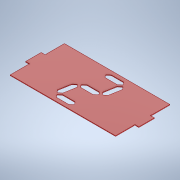
# Autodesk Inventor part: Cockpit_front_frame_cloth
Saved by Autodesk Inventor 2020 (Build 240168000, 168)
## iProperties
Created: 2022-04-01
Part Number: Cockpit_front_frame_cloth
Material: 一般
Document SubType Name: Modeling
Designer: Masato Kubotera
Density: 1 g/cm^3
Appearance: 滑らか - 赤
Author: Masato Kubotera
Autodesk Inventor part; units mm, degrees
ref_plane "XZ Plane" through (0, 0, 0) normal (0, 1, 0) x (-1, 0, 0)
ref_plane "XY Plane" through (0, 0, 0) normal (0, 0, 1) x (1, 0, 0)
derived "Cockpit_front_frame.ipt"
sketch "スケッチ2" plane through (0, 0, 0) normal (0, 1, 0) x (-1, 0, 0)
  line L0 (-28.5, -22.5) -> (88.5, -22.5) construction
  line L1 (88.5, -22.5) -> (88.5, -138.5)
  line L2 (88.5, -96) -> (-28.5, -96) construction
  line L3 (-28.5, -96) -> (-28.5, -22.5) construction
  line L4 (-28.5, -22.5) -> (88.5, -96) construction
  line L5 (88.5, -22.5) -> (-28.5, -96) construction
  line L6 (38.5, -101) -> (38.5, -133.5)
  line L7 (43.5, -138.5) -> (88.5, -138.5)
  line L8 (63.9, -63.85) -> (73.1, -63.85) construction
  line L9 (73.1, -63.85) -> (73.1, -77.65) construction
  line L10 (73.1, -77.65) -> (63.9, -77.65) construction
  line L11 (63.9, -77.65) -> (63.9, -63.85) construction
  line L12 (63.9, -63.85) -> (73.1, -77.65) construction
  line L13 (73.1, -63.85) -> (63.9, -77.65) construction
  line L14 (63.2, -63.2) -> (73.8, -63.2) construction
  line L15 (73.8, -63.2) -> (73.8, -78.3) construction
  line L16 (73.8, -78.3) -> (63.2, -78.3) construction
  line L17 (63.2, -78.3) -> (63.2, -63.2) construction
  line L18 (63.2, -63.2) -> (73.8, -78.3) construction
  line L19 (73.8, -63.2) -> (63.2, -78.3) construction
  line L20 (68.5, -63.2) -> (68.5, -78.3) construction
  line L21 (73.8, -70.75) -> (63.2, -70.75) construction
  line L22 (64.6349, -63.15) -> (72.3651, -63.15)
  line L23 (63.15, -64.6349) -> (63.15, -76.8651)
  line L24 (65.3349, -63.8) -> (71.6651, -63.8)
  line L25 (63.85, -65.2849) -> (63.85, -76.2151)
  arc A0 (64.6349, -63.15) -> (63.15, -64.6349) centre (63.8925, -63.8925) ccw
  arc A1 (65.3349, -63.8) -> (63.85, -65.2849) centre (64.5925, -64.5425) ccw
  arc A2 (73.85, -64.6349) -> (72.3651, -63.15) centre (73.1075, -63.8925) ccw
  arc A3 (73.15, -65.2849) -> (71.6651, -63.8) centre (72.4075, -64.5425) ccw
  line L26 (64.6349, -78.35) -> (72.3651, -78.35)
  line L27 (65.3349, -77.7) -> (71.6651, -77.7)
  arc A4 (63.85, -76.2151) -> (65.3349, -77.7) centre (64.5925, -76.9575) ccw
  arc A5 (63.15, -76.8651) -> (64.6349, -78.35) centre (63.8925, -77.6075) ccw
  arc A6 (72.3651, -78.35) -> (73.85, -76.8651) centre (73.1075, -77.6075) ccw
  arc A7 (71.6651, -77.7) -> (73.15, -76.2151) centre (72.4075, -76.9575) ccw
  line L28 (73.15, -65.2849) -> (73.15, -76.2151)
  line L29 (73.85, -64.6349) -> (73.85, -76.8651)
  line L30 (-23.5, -22.5) -> (-28.5, -27.5)
  line L31 (-28.5, -59.25) -> (88.5, -59.25) construction
  line L32 (30, -22.5) -> (30, -96) construction
  line L33 (-23.5, -96) -> (-28.5, -91)
  line L34 (-28.5, -27.5) -> (-28.5, -91)
  line L35 (-20.5, -24.5) -> (-25.5, -24.5) construction
  line L36 (-25.5, -24.5) -> (-25.5, -94) construction
  line L37 (-25.5, -94) -> (-20.5, -94) construction
  line L38 (-20.5, -94) -> (-20.5, -24.5) construction
  line L39 (-20.5, -24.5) -> (-25.5, -94) construction
  line L40 (-25.5, -24.5) -> (-20.5, -94) construction
  line L41 (-25.55, -46.7) -> (-20.45, -46.7)
  line L42 (-20.45, -46.7) -> (-20.45, -71.8)
  line L43 (-20.45, -71.8) -> (-25.55, -71.8)
  line L44 (-25.55, -71.8) -> (-25.55, -46.7)
  line L45 (-25.55, -46.7) -> (-20.45, -71.8) construction
  line L46 (-20.45, -46.7) -> (-25.55, -71.8) construction
  line L47 (-25.5, -46.75) -> (-20.5, -46.75) construction
  line L48 (-25.5, -71.75) -> (-20.5, -71.75) construction
  line L49 (-23, -24.5) -> (-23, -94) construction
  circle A8 centre (-23, -35) radius 3
  circle A9 centre (-23, -35) radius 1.6
  arc A10 (-24.0651, -46.7) -> (-25.55, -48.1849) centre (-24.8075, -47.4425) ccw
  arc A11 (-20.45, -48.1849) -> (-21.9349, -46.7) centre (-21.1925, -47.4425) ccw
  arc A12 (-25.55, -70.3151) -> (-24.0651, -71.8) centre (-24.8075, -71.0575) ccw
  arc A13 (-21.9349, -71.8) -> (-20.45, -70.3151) centre (-21.1925, -71.0575) ccw
  circle A14 centre (-23, -83.5) radius 3
  circle A15 centre (-23, -83.5) radius 1.6
  line L50 (33.5, -96) -> (38.5, -101)
  line L51 (-23.5, -96) -> (33.5, -96)
  line L52 (81, -42.5) -> (-20.5, -42.5) construction
  line L53 (-20.5, -42.5) -> (-20.5, -37.5) construction
  line L54 (-20.5, -37.5) -> (81, -37.5) construction
  line L55 (81, -37.5) -> (81, -42.5) construction
  line L56 (81, -42.5) -> (-20.5, -37.5) construction
  line L57 (-20.5, -42.5) -> (81, -37.5) construction
  line L58 (-20.5, -40) -> (81, -40) construction
  line L59 (30.25, -37.5) -> (30.25, -42.5) construction
  line L60 (5.25, -37.5) -> (5.25, -42.5) construction
  line L61 (55.3, -37.45) -> (5.2, -37.45)
  line L62 (5.2, -37.45) -> (5.2, -42.55)
  line L63 (5.2, -42.55) -> (55.3, -42.55)
  line L64 (55.3, -42.55) -> (55.3, -37.45)
  line L65 (55.3, -37.45) -> (5.2, -42.55) construction
  line L66 (5.2, -37.45) -> (55.3, -42.55) construction
  arc A16 (6.6849, -37.45) -> (5.2, -38.9349) centre (5.9425, -38.1925) ccw
  circle A17 centre (-2.25, -40) radius 3
  circle A18 centre (-2.25, -40) radius 1.6
  line L67 (55.25, -37.5) -> (55.25, -42.5) construction
  arc A19 (55.3, -38.9349) -> (53.8151, -37.45) centre (54.5575, -38.1925) ccw
  circle A20 centre (62.75, -40) radius 3
  circle A21 centre (62.75, -40) radius 1.6
  arc A22 (5.2, -41.0651) -> (6.6849, -42.55) centre (5.9425, -41.8075) ccw
  arc A23 (53.8151, -42.55) -> (55.3, -41.0651) centre (54.5575, -41.8075) ccw
  line L68 (-20.5, -89) -> (81, -89) construction
  line L69 (81, -89) -> (81, -94) construction
  line L70 (81, -94) -> (-20.5, -94) construction
  line L71 (-20.5, -94) -> (-20.5, -89) construction
  line L72 (-20.5, -89) -> (81, -94) construction
  line L73 (81, -89) -> (-20.5, -94) construction
  line L74 (-20.5, -91.5) -> (81, -91.5) construction
  line L75 (30.25, -89) -> (30.25, -94) construction
  line L76 (55.3, -91.55) -> (5.2, -91.55)
  line L77 (5.2, -91.55) -> (5.2, -88.95)
  line L78 (5.2, -88.95) -> (55.3, -88.95)
  line L79 (55.3, -88.95) -> (55.3, -91.55)
  line L80 (55.3, -91.55) -> (5.2, -88.95) construction
  line L81 (5.2, -91.55) -> (55.3, -88.95) construction
  line L82 (5.25, -89) -> (5.25, -91.5) construction
  line L83 (55.25, -89) -> (55.25, -91.5) construction
  line L84 (5.25, -90.25) -> (55.25, -90.25) construction
  arc A24 (7.3, -88.95) -> (5.2, -88.95) centre (6.25, -88.95) ccw
  arc A25 (55.3, -88.95) -> (53.2, -88.95) centre (54.25, -88.95) ccw
  arc A26 (5.2, -91.55) -> (7.3, -91.55) centre (6.25, -91.55) ccw
  arc A27 (53.2, -91.55) -> (55.3, -91.55) centre (54.25, -91.55) ccw
  circle A28 centre (-2.5, -91.5) radius 3
  circle A29 centre (-2.5, -91.5) radius 1.6
  circle A30 centre (62.5, -91.5) radius 3 construction
  circle A31 centre (62.5, -91.5) radius 1.6 construction
  line L85 (-23.5, -22.5) -> (63.7651, -22.5)
  line L86 (65.25, -21.0151) -> (65.25, -17.5)
  line L87 (65.25, -17.5) -> (73.25, -17.5)
  line L88 (73.25, -17.5) -> (73.25, -21.0151)
  line L89 (81, -22.5) -> (81, -17.5)
  line L90 (88.5, -22.5) -> (88.5, -20)
  line L91 (81, -17.5) -> (86, -17.5)
  line L92 (86, -17.5) -> (88.5, -20)
  line L93 (69.25, -17.5) -> (69.25, -22.5) construction
  arc A32 (63.7651, -22.5) -> (65.25, -21.0151) centre (64.5075, -21.7575) ccw
  arc A33 (73.25, -21.0151) -> (74.7349, -22.5) centre (73.9925, -21.7575) ccw
  arc A34 (79.5151, -22.5) -> (81, -21.0151) centre (80.2575, -21.7575) ccw
  line L94 (-15.5, -89) -> (-15.5, -69) construction
  line L95 (-15.5, -69) -> (64.5, -69) construction
  line L96 (64.5, -69) -> (64.5, -89) construction
  line L97 (45.5, -84) -> (-16.5, -84)
  line L98 (-18.5, -82) -> (-18.5, -63.3955)
  line L99 (-16.5, -61.3955) -> (45.5, -61.3955)
  line L100 (47.5, -63.3955) -> (47.5, -82)
  line L101 (47.5, -84) -> (-18.5, -61.3955) construction
  line L102 (-18.5, -84) -> (47.5, -61.3955) construction
  arc A35 (-16.5, -61.3955) -> (-18.5, -63.3955) centre (-16.5, -63.3955) ccw
  arc A36 (-18.5, -82) -> (-16.5, -84) centre (-16.5, -82) ccw
  arc A37 (45.5, -84) -> (47.5, -82) centre (45.5, -82) ccw
  arc A38 (47.5, -63.3955) -> (45.5, -61.3955) centre (45.5, -63.3955) ccw
  line L103 (38.5, -133.5) -> (43.5, -138.5)
  line L104 (46, -131) -> (41, -131) construction
  line L105 (41, -131) -> (41, -96) construction
  line L106 (41, -96) -> (46, -96) construction
  line L107 (46, -96) -> (46, -131) construction
  line L108 (46, -131) -> (41, -96) construction
  line L109 (41, -131) -> (46, -96) construction
  line L110 (43.5, -96) -> (43.5, -131) construction
  line L111 (41, -113.5) -> (46, -113.5) construction
  line L112 (43.5, -107.5) -> (46, -107.5) construction
  line L113 (43.45, -107.45) -> (46.05, -107.45)
  line L114 (46.05, -107.45) -> (46.05, -119.55)
  line L115 (46.05, -119.55) -> (43.45, -119.55)
  line L116 (43.45, -119.55) -> (43.45, -107.45)
  line L117 (43.45, -107.45) -> (46.05, -119.55) construction
  line L118 (46.05, -107.45) -> (43.45, -119.55) construction
  arc A39 (46.05, -109.55) -> (46.05, -107.45) centre (46.05, -108.5) ccw
  arc A40 (44.9349, -107.45) -> (43.45, -108.9349) centre (44.1925, -108.1925) ccw
  line L119 (43.5, -119.5) -> (46, -119.5) construction
  arc A41 (46.05, -119.55) -> (46.05, -117.45) centre (46.05, -118.5) ccw
  arc A42 (43.45, -118.0651) -> (44.9349, -119.55) centre (44.1925, -118.8075) ccw
  line L120 (44.75, -107.5) -> (44.75, -119.5) construction
  circle A43 centre (43.5, -125.5) radius 3 construction
  circle A44 centre (43.5, -125.5) radius 1.6 construction
  circle A45 centre (43.5, -101.5) radius 3
  circle A46 centre (43.5, -101.5) radius 1.6
  circle A47 centre (-13.5, -55) radius 2
  line L121 (41, -131) -> (79.8645, -131) construction
  line L122 (79.8645, -131) -> (79.8645, -136) construction
  line L123 (79.8645, -136) -> (41, -136) construction
  line L124 (41, -136) -> (41, -131) construction
  line L125 (41, -131) -> (79.8645, -136) construction
  line L126 (79.8645, -131) -> (41, -136) construction
  line L127 (41, -133.5) -> (79.8645, -133.5) construction
  line L128 (60.4322, -131) -> (60.4322, -136) construction
  line L129 (60.4322, -133.5) -> (60.4322, -131) construction
  line L130 (52.8822, -130.95) -> (67.9822, -130.95)
  line L131 (67.9822, -130.95) -> (67.9822, -133.55)
  line L132 (67.9822, -133.55) -> (52.8822, -133.55)
  line L133 (52.8822, -133.55) -> (52.8822, -130.95)
  line L134 (52.8822, -130.95) -> (67.9822, -133.55) construction
  line L135 (67.9822, -130.95) -> (52.8822, -133.55) construction
  line L136 (52.9322, -131) -> (52.9322, -133.5) construction
  arc A48 (54.9822, -130.95) -> (52.8822, -130.95) centre (53.9322, -130.95) ccw
  arc A49 (52.8822, -132.0651) -> (54.3672, -133.55) centre (53.6247, -132.8075) ccw
  arc A50 (67.9822, -130.95) -> (65.8822, -130.95) centre (66.9322, -130.95) ccw
  arc A51 (66.4973, -133.55) -> (67.9822, -132.0651) centre (67.2398, -132.8075) ccw
  line L137 (67.9322, -131) -> (67.9322, -133.5) construction
  line L138 (52.9322, -132.25) -> (67.9322, -132.25) construction
  circle A52 centre (74.4322, -133.5) radius 1.6 construction
  circle A53 centre (74.4322, -133.5) radius 3 construction
  circle A54 centre (46.4322, -133.5) radius 1.6
  circle A55 centre (46.4322, -133.5) radius 3
  line L139 (50.5, -96.5) -> (79, -96.5)
  line L140 (81, -98.5) -> (81, -126.5)
  line L141 (79, -128.5) -> (50.5, -128.5)
  line L142 (48.5, -126.5) -> (48.5, -98.5)
  line L143 (48.5, -96.5) -> (81, -128.5) construction
  line L144 (81, -96.5) -> (48.5, -128.5) construction
  arc A56 (50.5, -96.5) -> (48.5, -98.5) centre (50.5, -98.5) ccw
  arc A57 (48.5, -126.5) -> (50.5, -128.5) centre (50.5, -126.5) ccw
  arc A58 (79, -128.5) -> (81, -126.5) centre (79, -126.5) ccw
  arc A59 (81, -98.5) -> (79, -96.5) centre (79, -98.5) ccw
  line L145 (81, -91.6746) -> (86, -91.6746) construction
  line L146 (86, -91.6746) -> (86, -136) construction
  line L147 (86, -136) -> (81, -136) construction
  line L148 (81, -136) -> (81, -91.6746) construction
  line L149 (81, -91.6746) -> (86, -136) construction
  line L150 (86, -91.6746) -> (81, -136) construction
  line L151 (83.5, -91.6746) -> (83.5, -136) construction
  circle A60 centre (83.5, -94.1746) radius 1.475
  circle A61 centre (83.5, -99.1746) radius 1.475
  circle A62 centre (83.5, -104.1746) radius 1.475
  circle A63 centre (83.5, -133.5) radius 1.6
  arc A64 (86, -91.6746) -> (81, -91.6746) centre (83.5, -133.5) ccw construction
  arc A65 (86.0112, -91.5751) -> (80.9888, -91.5751) centre (83.5, -133.5) ccw construction
  line L152 (88.5, -133.5) -> (83.5, -138.5)
  arc A66 (81, -131) -> (86, -136) centre (83.5, -133.5) ccw construction
  line L153 (86, -91.5) -> (81, -91.5) construction
  circle A67 centre (83.5, -133.5) radius 3
  line L154 (77.125, -22.5) -> (77.125, -27.147) construction
  line L155 (61.375, -22.5) -> (61.375, -27.147) construction
  line L156 (65.25, -22.5) -> (73.25, -22.5)
  line L157 (-18.5, -29.5) -> (-18.5, -31.2215)
  line L158 (-16.5, -33.2215) -> (45.5, -33.2215)
  line L159 (47.5, -31.2215) -> (47.5, -29.5)
  line L160 (45.5, -27.5) -> (-16.5, -27.5)
  arc A68 (-16.5, -27.5) -> (-18.5, -29.5) centre (-16.5, -29.5) ccw
  arc A69 (-18.5, -31.2215) -> (-16.5, -33.2215) centre (-16.5, -31.2215) ccw
  arc A70 (45.5, -33.2215) -> (47.5, -31.2215) centre (45.5, -31.2215) ccw
  arc A71 (47.5, -29.5) -> (45.5, -27.5) centre (45.5, -29.5) ccw
  line L161 (81, -66.9105) -> (86, -66.9105) construction
  line L162 (86, -66.9105) -> (86, -46.9105) construction
  line L163 (86, -46.9105) -> (81, -46.9105) construction
  line L164 (81, -46.9105) -> (81, -66.9105) construction
  line L165 (81, -66.9105) -> (86, -46.9105) construction
  line L166 (86, -66.9105) -> (81, -46.9105) construction
  line L167 (81, -22.5) -> (81, -28.5) construction
  line L168 (81, -28.5) -> (57.5, -28.5) construction
  line L169 (57.5, -28.5) -> (57.5, -22.5) construction
  line L170 (74.7349, -22.5) -> (79.5151, -22.5) construction
  line L171 (74.7349, -22.5) -> (79.5151, -22.5)
  point P0 (0, 0)
  point P1 (30, -59.25)
  point P2 (-25.7227, -96)
  point P3 (68.5, -70.75)
  point P4 (63.15, -63.15)
  point P5 (63.85, -63.8)
  point P6 (-23, -59.25)
  point P7 (30.25, -40)
  point P8 (30.25, -91.5)
  point P9 (30.25, -90.25)
  point P10 (30.25, -90.25)
  point P11 (52.5, -22)
  point P12 (14.5, -72.6978)
  point P13 (-18.5, -61)
  point P14 (47.5, -61)
  point P15 (43.5, -113.5)
  point P16 (44.75, -113.5)
  point P17 (60.4322, -132.25)
  point P18 (64.75, -112.5)
  point P19 (83.5, -113.8373)
  point P20 (-18.5, -33.2215)
  point P21 (47.5, -27.5)
  point P22 (-18.5, -27.5)
  point P23 (83.5, -56.9105)
  point P24 (69.25, -28.5)
  point P25 (73.7349, -22.5)
  point P26 (72.25, -21.0151)
  point P27 (64.4973, -133.55)
  point P28 (63.8822, -130.95)
  point P29 (65.9822, -132.0651)
  point P30 (41.45, -118.0651)
  point P31 (44.05, -117.45)
  point P32 (42.9349, -119.55)
  point P33 (-26.05, -70.3151)
  point P34 (-22.4349, -46.7)
  point P35 (-20.95, -48.1849)
  point P36 (-20.95, -70.3151)
  point P37 (-22.4349, -71.8)
  point P38 (-24.5651, -71.8)
  point P39 (54.05, -59.5651)
  point P40 (52.5651, -61.05)
  point P41 (5.4349, -61.05)
  point P42 (3.95, -59.5651)
  point P43 (52.5651, -55.95)
  point P44 (54.05, -57.4349)
  point P45 (51.95, -88.45)
  point P46 (51.95, -91.05)
  point P47 (6.05, -91.05)
  point P48 (80.4349, -79.8)
  point P49 (78.95, -78.3151)
  point P50 (72.25, -22.5)
  point P51 (73.25, -21.0151)
  point P52 (66.4973, -133.55)
  point P53 (43.45, -118.0651)
  point P54 (44.9349, -119.55)
  point P55 (-25.55, -70.3151)
  point P56 (-21.9349, -46.7)
  point P57 (-21.9349, -71.8)
  point P58 (-24.0651, -71.8)
  point P59 (55.3, -41.0651)
  point P60 (53.8151, -42.55)
  point P61 (6.6849, -42.55)
  point P62 (5.2, -41.0651)
  point P63 (53.8151, -37.45)
  point P64 (55.3, -38.9349)
  point P65 (53.2, -88.95)
  point P66 (53.2, -91.55)
sketch "スケッチ3" plane through (20.5, 0, 0) normal (1, 0, 0) x (0, 1, 0)
  line L0 (-135, -24.5) -> (0, -24.5)
  line L1 (0, -24.5) -> (0, -94)
  line L2 (0, -94) -> (-135, -94)
  line L3 (-135, -94) -> (-135, -24.5)
  line L4 (-135, -24.5) -> (0, -94) construction
  line L5 (0, -24.5) -> (-135, -94) construction
  line L6 (0, -71.75) -> (5, -71.75)
  line L7 (5, -71.75) -> (5, -46.75)
  line L8 (5, -46.75) -> (0, -46.75)
  line L9 (0, -59.25) -> (-135, -59.25) construction
  line L10 (-67.5, -94) -> (-67.5, -24.5)
  arc A0 (1.4849, -71.75) -> (0, -73.2349) centre (0.7425, -72.4925) ccw
  arc A1 (0, -45.2651) -> (1.4849, -46.75) centre (0.7425, -46.0075) ccw
  line L11 (-128, -89) -> (-7, -89)
  line L12 (-5, -87) -> (-5, -44.5)
  line L13 (-7, -42.5) -> (-128, -42.5)
  line L14 (-130, -44.5) -> (-130, -87)
  line L15 (-130, -89) -> (-5, -42.5) construction
  line L16 (-5, -89) -> (-130, -42.5) construction
  line L17 (-128, -29.5) -> (-7, -29.5)
  line L18 (-5, -31.5) -> (-5, -35.5)
  line L19 (-7, -37.5) -> (-128, -37.5)
  line L20 (-130, -35.5) -> (-130, -31.5)
  line L21 (-130, -29.5) -> (-5, -37.5) construction
  line L22 (-5, -29.5) -> (-130, -37.5) construction
  arc A2 (-7, -89) -> (-5, -87) centre (-7, -87) ccw
  arc A3 (-5, -44.5) -> (-7, -42.5) centre (-7, -44.5) ccw
  arc A4 (-128, -42.5) -> (-130, -44.5) centre (-128, -44.5) ccw
  arc A5 (-130, -87) -> (-128, -89) centre (-128, -87) ccw
  arc A6 (-130, -35.5) -> (-128, -37.5) centre (-128, -35.5) ccw
  arc A7 (-7, -37.5) -> (-5, -35.5) centre (-7, -35.5) ccw
  arc A8 (-5, -31.5) -> (-7, -29.5) centre (-7, -31.5) ccw
  arc A9 (-128, -29.5) -> (-130, -31.5) centre (-128, -31.5) ccw
  point P0 (0, 0)
  point P1 (-67.5, -59.25)
  point P2 (0, -24.5)
  point P3 (0, -42.5)
  point P4 (0, -42.5)
  point P5 (0, -42.5)
  point P6 (0, -37.5)
  point P7 (0, -37.5)
  point P8 (0, -37.5)
  point P9 (-67.5, -65.75)
  point P10 (-67.5, -33.5)
  point P11 (0, -46.75)
  point P12 (0, -45.2651)
  point P13 (1.4849, -46.75)
  point P14 (-67.5, -42.5)
  point P15 (-67.5, -89)
  point P16 (-67.5, -29.5)
  point P17 (-67.5, -37.5)
ref_plane "作業平面1" through (10, 0, 0) normal (1, 0, 0) x (0, 1, 0)
sketch "スケッチ4" plane through (10, 0, 0) normal (1, 0, 0) x (0, 1, 0)
  line L0 (-135, -24.5) -> (0, -24.5)
  line L1 (0, -24.5) -> (0, -47.7651)
  line L2 (0, -94) -> (-135, -94)
  line L3 (-135, -94) -> (-135, -70.7349)
  line L4 (0, -49.25) -> (5, -49.25)
  line L5 (5, -49.25) -> (5, -69.25)
  line L6 (5, -69.25) -> (0, -69.25)
  arc A0 (0, -47.7651) -> (1.4849, -49.25) centre (0.7425, -48.5075) ccw
  line L7 (5, -71.75) -> (5, -46.75) projected
  line L8 (0, -59.25) -> (-135, -59.25) construction
  arc A1 (1.4849, -69.25) -> (0, -70.7349) centre (0.7425, -69.9925) ccw
  line L9 (-67.5, -94) -> (-67.5, -24.5) construction
  line L10 (-135, -49.25) -> (-140, -49.25)
  line L11 (-140, -49.25) -> (-140, -69.25)
  line L12 (-140, -69.25) -> (-135, -69.25)
  arc A2 (-136.4849, -49.25) -> (-135, -47.7651) centre (-135.7425, -48.5075) ccw
  arc A3 (-135, -70.7349) -> (-136.4849, -69.25) centre (-135.7425, -69.9925) ccw
  line L13 (-75.9814, -35.4371) -> (-73.9871, -37.8138)
  line L14 (-73.6833, -33.5087) -> (-71.6889, -35.8855)
  line L15 (-70.4337, -29.4767) -> (-73.56, -32.0999)
  line L16 (-77.3902, -35.3138) -> (-80.5165, -37.9371)
  line L17 (-69.7909, -29.2427) -> (-54.7292, -29.2427)
  line L18 (-55.2184, -36.0087) -> (-52.0921, -33.3855)
  line L19 (-53.9632, -29.5999) -> (-51.9688, -31.9767)
  line L20 (-70.9229, -36.2427) -> (-55.8612, -36.2427)
  line L21 (-73.7683, -38.6303) -> (-76.3837, -53.4632)
  line L22 (-76.7258, -54.0556) -> (-79.852, -56.6788)
  line L23 (-81.2609, -56.5556) -> (-83.2552, -54.1788)
  line L24 (-80.8585, -38.5295) -> (-83.474, -53.3624)
  line L25 (-76.6242, -34.6711) -> (-80.6181, -57.3216) construction
  line L26 (-51.326, -32.7427) -> (-74.326, -32.7427) construction
  arc A4 (-75.9814, -35.4371) -> (-77.3902, -35.3138) centre (-76.7474, -36.0799) ccw
  arc A5 (-73.7683, -38.6303) -> (-73.9871, -37.8138) centre (-74.7531, -38.4566) ccw
  arc A6 (-76.7258, -54.0556) -> (-76.3837, -53.4632) centre (-77.3686, -53.2895) ccw
  arc A7 (-81.2609, -56.5556) -> (-79.852, -56.6788) centre (-80.4948, -55.9128) ccw
  arc A8 (-83.474, -53.3624) -> (-83.2552, -54.1788) centre (-82.4892, -53.5361) ccw
  arc A9 (-80.5165, -37.9371) -> (-80.8585, -38.5295) centre (-79.8737, -38.7031) ccw
  arc A10 (-55.8612, -36.2427) -> (-55.2184, -36.0087) centre (-55.8612, -35.2427) ccw
  arc A11 (-52.0921, -33.3855) -> (-51.9688, -31.9767) centre (-52.7349, -32.6194) ccw
  arc A12 (-53.9632, -29.5999) -> (-54.7292, -29.2427) centre (-54.7292, -30.2427) ccw
  arc A13 (-69.7909, -29.2427) -> (-70.4337, -29.4767) centre (-69.7909, -30.2427) ccw
  arc A14 (-73.56, -32.0999) -> (-73.6833, -33.5087) centre (-72.9172, -32.866) ccw
  arc A15 (-71.6889, -35.8855) -> (-70.9229, -36.2427) centre (-70.9229, -35.2427) ccw
  line L27 (-135, -47.7651) -> (-135, -24.5)
  line L28 (-135, -70.7349) -> (-135, -47.7651) construction
  line L29 (0, -47.7651) -> (0, -70.7349) construction
  line L30 (0, -70.7349) -> (0, -94)
  line L31 (-49.0652, -35.4371) -> (-47.0708, -37.8138)
  line L32 (-50.474, -35.3138) -> (-53.6003, -37.9371)
  arc A16 (-49.0652, -35.4371) -> (-50.474, -35.3138) centre (-49.8312, -36.0799) ccw
  line L33 (-53.9423, -38.5295) -> (-56.5577, -53.3624)
  arc A17 (-53.6003, -37.9371) -> (-53.9423, -38.5295) centre (-52.9575, -38.7031) ccw
  arc A18 (-46.8521, -38.6303) -> (-47.0708, -37.8138) centre (-47.8369, -38.4566) ccw
  line L34 (-46.8521, -38.6303) -> (-49.4675, -53.4632)
  arc A19 (-49.8095, -54.0556) -> (-49.4675, -53.4632) centre (-50.4523, -53.2895) ccw
  line L35 (-49.8095, -54.0556) -> (-52.9358, -56.6788)
  arc A20 (-54.3447, -56.5556) -> (-52.9358, -56.6788) centre (-53.5786, -55.9128) ccw
  line L36 (-54.3447, -56.5556) -> (-56.339, -54.1788)
  arc A21 (-56.5577, -53.3624) -> (-56.339, -54.1788) centre (-55.5729, -53.5361) ccw
  line L37 (-80.6553, -61.9444) -> (-78.661, -64.3212)
  line L38 (-82.0642, -61.8212) -> (-85.1905, -64.4444)
  arc A22 (-80.6553, -61.9444) -> (-82.0642, -61.8212) centre (-81.4214, -62.5872) ccw
  line L39 (-85.5325, -65.0368) -> (-88.1479, -79.8697)
  arc A23 (-85.1905, -64.4444) -> (-85.5325, -65.0368) centre (-84.5477, -65.2105) ccw
  arc A24 (-78.4423, -65.1376) -> (-78.661, -64.3212) centre (-79.4271, -64.9639) ccw
  line L40 (-78.4423, -65.1376) -> (-81.0577, -79.9705)
  arc A25 (-81.3997, -80.5629) -> (-81.0577, -79.9705) centre (-82.0425, -79.7969) ccw
  line L41 (-81.3997, -80.5629) -> (-84.526, -83.1862)
  arc A26 (-85.9348, -83.0629) -> (-84.526, -83.1862) centre (-85.1688, -82.4201) ccw
  line L42 (-85.9348, -83.0629) -> (-87.9292, -80.6862)
  arc A27 (-88.1479, -79.8697) -> (-87.9292, -80.6862) centre (-87.1631, -80.0434) ccw
  line L43 (-53.7391, -61.9444) -> (-51.7448, -64.3212)
  line L44 (-55.148, -61.8212) -> (-58.2742, -64.4444)
  arc A28 (-53.7391, -61.9444) -> (-55.148, -61.8212) centre (-54.5052, -62.5872) ccw
  line L45 (-58.6163, -65.0368) -> (-61.2317, -79.8697)
  arc A29 (-58.2742, -64.4444) -> (-58.6163, -65.0368) centre (-57.6314, -65.2105) ccw
  arc A30 (-51.526, -65.1376) -> (-51.7448, -64.3212) centre (-52.5108, -64.9639) ccw
  line L46 (-51.526, -65.1376) -> (-54.1415, -79.9705)
  arc A31 (-54.4835, -80.5629) -> (-54.1415, -79.9705) centre (-55.1263, -79.7969) ccw
  line L47 (-54.4835, -80.5629) -> (-57.6098, -83.1862)
  arc A32 (-59.0186, -83.0629) -> (-57.6098, -83.1862) centre (-58.2526, -82.4201) ccw
  line L48 (-59.0186, -83.0629) -> (-61.0129, -80.6862)
  arc A33 (-61.2317, -79.8697) -> (-61.0129, -80.6862) centre (-60.2469, -80.0434) ccw
  line L49 (-74.4649, -55.75) -> (-59.4032, -55.75)
  arc A34 (-74.4649, -55.75) -> (-75.1077, -55.984) centre (-74.4649, -56.75) ccw
  line L50 (-75.1077, -55.984) -> (-78.234, -58.6072)
  arc A35 (-78.234, -58.6072) -> (-78.3572, -60.016) centre (-77.5912, -59.3733) ccw
  line L51 (-78.3572, -60.016) -> (-76.3629, -62.3928)
  arc A36 (-76.3629, -62.3928) -> (-75.5968, -62.75) centre (-75.5968, -61.75) ccw
  line L52 (-75.5968, -62.75) -> (-60.5351, -62.75)
  arc A37 (-60.5351, -62.75) -> (-59.8923, -62.516) centre (-60.5351, -61.75) ccw
  line L53 (-59.8923, -62.516) -> (-56.766, -59.8928)
  arc A38 (-56.766, -59.8928) -> (-56.6428, -58.484) centre (-57.4088, -59.1267) ccw
  line L54 (-58.6371, -56.1072) -> (-56.6428, -58.484)
  arc A39 (-58.6371, -56.1072) -> (-59.4032, -55.75) centre (-59.4032, -56.75) ccw
  line L55 (-79.1388, -82.2573) -> (-64.0771, -82.2573)
  arc A40 (-79.1388, -82.2573) -> (-79.7816, -82.4913) centre (-79.1388, -83.2573) ccw
  line L56 (-79.7816, -82.4913) -> (-82.9079, -85.1145)
  arc A41 (-82.9079, -85.1145) -> (-83.0312, -86.5233) centre (-82.2651, -85.8806) ccw
  line L57 (-83.0312, -86.5233) -> (-81.0368, -88.9001)
  arc A42 (-81.0368, -88.9001) -> (-80.2708, -89.2573) centre (-80.2708, -88.2573) ccw
  line L58 (-80.2708, -89.2573) -> (-65.2091, -89.2573)
  arc A43 (-65.2091, -89.2573) -> (-64.5663, -89.0233) centre (-65.2091, -88.2573) ccw
  line L59 (-64.5663, -89.0233) -> (-61.44, -86.4001)
  arc A44 (-61.44, -86.4001) -> (-61.3167, -84.9913) centre (-62.0828, -85.634) ccw
  line L60 (-63.3111, -82.6145) -> (-61.3167, -84.9913)
  arc A45 (-63.3111, -82.6145) -> (-64.0771, -82.2573) centre (-64.0771, -83.2573) ccw
  line L61 (-66.934, -55.75) -> (-68.066, -62.75) construction
  point P0 (0, 0)
  point P1 (1.4849, -69.25)
  point P2 (-135, -47.7651)
  point P3 (0, -70.7349)
  point P4 (-135, -49.25)
  point P5 (0, -69.25)
  point P6 (-80.7953, -38.1711)
  point P7 (-73.6873, -38.1711)
  point P8 (-71.3892, -36.2427)
  point P9 (-70.1549, -29.2427)
  point P10 (-54.2629, -29.2427)
  point P11 (-55.4972, -36.2427)
  point P12 (-76.447, -53.8216)
  point P13 (-83.5549, -53.8216)
  point P14 (-67.5, -59.25)
  point P15 (-49.708, -34.6711)
  point P16 (-46.7711, -38.1711)
  point P17 (-53.8791, -38.1711)
  point P18 (-56.6387, -53.8216)
  point P19 (-49.5307, -53.8216)
  point P20 (-53.7019, -57.3216)
  point P21 (-81.2981, -61.1784)
  point P22 (-78.3613, -64.6784)
  point P23 (-85.4693, -64.6784)
  point P24 (-88.2289, -80.3289)
  point P25 (-81.1209, -80.3289)
  point P26 (-85.292, -83.8289)
  point P27 (-54.3819, -61.1784)
  point P28 (-51.4451, -64.6784)
  point P29 (-58.553, -64.6784)
  point P30 (-61.3127, -80.3289)
  point P31 (-54.2047, -80.3289)
  point P32 (-58.3758, -83.8289)
  point P33 (-58.9368, -55.75)
  point P34 (-74.8289, -55.75)
  point P35 (-79, -59.25)
  point P36 (-76.0632, -62.75)
  point P37 (-60.1711, -62.75)
  point P38 (-56, -59.25)
  point P39 (-63.6108, -82.2573)
  point P40 (-79.5028, -82.2573)
  point P41 (-83.674, -85.7573)
  point P42 (-80.7371, -89.2573)
  point P43 (-64.8451, -89.2573)
  point P44 (-60.674, -85.7573)
  point P45 (-67.5, -59.25)
  dimension "d2" = 1.05
  dimension "d3" = 20
  dimension "d41" = 3
  dimension "d42" = 7
  dimension "d43" = 7
  dimension "d44" = 23
  dimension "d45" = 23
  dimension "d70" = 1
  dimension "d71" = 1
  dimension "d102" = 10
  dimension "d105" = 26.9162
  dimension "d108" = 26.9162
  dimension "d113" = 26.9162
  constraints: 118 end point, 93 point on circle, 91 point on line, 46 centre point, 24 tangent, 16 parallel, 13 symmetric about line, 10 equal radius, 8 perpendicular, 6 collinear, 6 midpoint, 3 horizontal, 2 coincident, 188 other
  measures "d2" radius of A0
  measures "d3" distance of L4.end L5.end
  measures "d41" distance between parallel lines of L13 L14
  measures "d42" distance between parallel lines of L20 L17
  measures "d43" distance between parallel lines of L21 L24
  measures "d44" distance of L26.start L26.end
  measures "d45" distance of L25.start L25.end
  measures "d70" radius of A4
  measures "d71" radius of A10
  measures "d102" angle of L9 L25
  measures "d105" distance of L13.start L31.start
  measures "d108" distance of L13.start L37.start
  measures "d113" distance of L17.start L49.start
extrude "押し出し1" add sketch "スケッチ4" along normal blind 0.75 contours L0 L1 A0 L4 L5 L6 A1 L30 L2 L3 A3 L12 L11 L10 A2 L27 | L13 A5 L21 A6 L22 A7 L23 A8 L24 A9 L16 A4 | L43 A30 L46 A31 L47 A32 L48 A33 L45 A29 L44 A28
equation "\"d43\" = d42"
